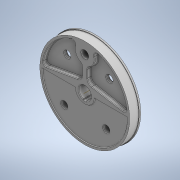
# Autodesk Inventor part: МТ10-3.00.00.02
Saved by Autodesk Inventor 2021 (Build 250183000, 183)
## iProperties
Created: 2022-06-08
Part Number: МТ10-3.00.00.02
Material: Типовые
Document SubType Name: Modeling
Designer: u
Density: 1 g/cm^3
Appearance: По умолчанию
Description: Диск
Mass: 2664.31 g
Surface Area: 2672.83 cm^2
Volume: 2664.31 cm^3
Author: u
Title: Диск
Autodesk Inventor part; units mm, degrees
ref_plane "YZ Plane" through (0, 0, 0) normal (1, 0, 0) x (0, 1, 0)
ref_plane "XZ Plane" through (0, 0, 0) normal (0, 1, 0) x (-1, 0, 0)
ref_plane "XY Plane" through (0, 0, 0) normal (0, 0, 1) x (1, 0, 0)
sketch "Эскиз1" plane through (0, 0, 0) normal (0, 0, 1) x (1, 0, 0)
  circle A0 centre (0, 0) radius 172
  circle A1 centre (0, 0) radius 162
  arc A2 (-36.4522, 138.735) -> (36.4522, 138.735) centre (0, 128) ccw
  arc A3 (-36.4522, 138.735) -> (-51.8004, 153.495) centre (-47.9634, 142.125) ccw
  circle A4 centre (0, 0) radius 38
  line L0 (26.527, 33.9088) -> (145.8715, 12.8651)
  line L1 (-240.8, 0) -> (240.8, 0) projected
  arc A5 (145.8715, 12.8651) -> (159.7917, 26.6575) centre (147.9553, 24.6828) ccw
  arc A6 (10, 53.6049) -> (26.527, 33.9088) centre (30, 53.6049) ccw
  line L2 (10, 53.6049) -> (10, 83.1001)
  arc A7 (16.72, 93.8761) -> (10, 83.1001) centre (22, 83.1001) ccw
  arc A8 (51.8004, 153.495) -> (36.4522, 138.735) centre (47.9634, 142.125) ccw
  arc A9 (-159.7917, 26.6575) -> (-145.8715, 12.8651) centre (-147.9553, 24.6828) ccw
  line L3 (-145.8715, 12.8651) -> (-26.527, 33.9088)
  arc A10 (-26.527, 33.9088) -> (-10, 53.6049) centre (-30, 53.6049) ccw
  line L4 (-10, 53.6049) -> (-10, 83.1001)
  arc A11 (-10, 83.1001) -> (-16.72, 93.8761) centre (-22, 83.1001) ccw
  line L5 (0, 0) -> (-80.6102, 80.6102)
  line L6 (6.4, -23.1309) -> (6.4, -26.9)
  line L7 (6.4, -26.9) -> (-6.4, -26.9)
  line L8 (-6.4, -26.9) -> (-6.4, -23.1309)
  arc A12 (6.4, -23.1309) -> (-6.4, -23.1309) centre (0, 0) ccw
  point P0 (-80.6102, -80.6102)
  point P1 (80.6102, -80.6102)
  point P2 (80.6102, 80.6102)
  point P3 (0, -26.9)
  point P4 (162, 0)
  point P5 (38, 0)
  point P6 (-38, 0)
  point P7 (-162, 0)
  dimension "d1" = 344
  dimension "d7" = 324
  dimension "d10" = 38
  dimension "d12" = 12
  dimension "d14" = 76
  dimension "d15" = 10
  dimension "d16" = 12
  dimension "d20" = 20
  dimension "d27" = 10
  dimension "d28" = 29.4952
  dimension "d29" = 12
  dimension "d31" = 12
  dimension "d33" = 12
  dimension "d36" = 10
  dimension "d37" = 20
  dimension "d38" = 12
  dimension "d39" = 45
  dimension "d40" = 114
  dimension "d43" = 360
  dimension "d45" = 26.9
  dimension "d46" = 12.8
  dimension "d47" = 24
  dimension "d61" = 128
  constraints: 26 point on circle, 16 end point, 16 tangent, 13 centre point, 4 coincident, 4 horizontal alignment, 3 vertical, 2 vertical alignment, 1 midpoint, 1 parallel, 5 other
  measures "d1" diameter of A0
  measures "d7" diameter of A1
  measures "d10" radius of A2
  measures "d12" radius of A3
  measures "d14" diameter of A4
  measures "d15" angle of L1 L0
  measures "d16" radius of A5
  measures "d20" radius of A6
  measures "d27" distance from line of L5.start L2
  measures "d28" distance of L2.start L2.end
  measures "d29" radius of A7
  measures "d31" radius of A8
  measures "d33" radius of A9
  measures "d36" angle of L1 L3
  measures "d37" radius of A10
  measures "d38" radius of A11
  measures "d39" angle of L1 L5
  measures "d40" distance of L5.start L5.end
  measures "d45" distance between parallel lines of L1 L7
  measures "d46" distance of L6.end L7.end
  measures "d47" radius of A12
  measures "d61" distance of L5.start A2.centre
extrude "Выдавливание1" add sketch "Эскиз1" along normal mid plane 12 contours A5 L0 A6 L2 A7 A2 A8 A1 | A1 A3 A2 A11 L4 A10 L3 A9
extrude "Выдавливание2" add sketch "Эскиз1" along normal mid plane 36 contours A1 L1 A4
extrude "Выдавливание3" add sketch "Эскиз1" along normal mid plane 40 contours L1 A1 A0 | A0 L1 A1 | L1 A4 L5 L3 A10 L4 A11 A2 A7 L2 A6 L0 A5 A1 | A1 A9 L3 L5 A4 L1 | L1 A12 L5 A4 | A4 L1 A12 L8 L7 L6 | A4 L5 A12 L1 | A8 A2 A3 A1
hole "Отверстие2" at (-80.6102, 80.6102, 0) at (-80.6102, -80.6102, 0) at (80.6102, -80.6102, 0) at (80.6102, 80.6102, 0) direction (0, 0, -1) diameter 24 end through all both
sketch "Эскиз2" plane through (0, 0, 20) normal (0, 0, 1) x (1, 0, 0)
  arc A0 (16.72, 93.8761) -> (36.4522, 138.735) centre (0, 128) ccw projected
  point P0 (0, 0)
  constraints: 1 coincident
hole "Отверстие3" at (0, 128, 20) direction (0, 0, -1) diameter 30 end through all
sketch "Эскиз4" plane through (0, 0, 0) normal (1, 0, 0) x (0, 1, 0)
  line L0 (172, -20) -> (172, 20) projected
  line L1 (172, -14) -> (174.5, -14)
  line L2 (174.5, -14) -> (174.5, -20)
  line L3 (174.5, -20) -> (172, -20)
  line L4 (0, 5.1312) -> (0, -5.1312)
  point P0 (0, 0)
  point P1 (0, 0)
  dimension "d80" = 2.5
  dimension "d81" = 6
  dimension "d82" = 10.2624
  constraints: 8 end point, 2 perpendicular, 1 coincident, 1 horizontal, 1 midpoint, 1 point on line, 1 vertical
  measures "d80" distance of L1.start L1.end
  measures "d81" distance of L1.end L2.end
  measures "d82" distance of L4.start L4.end
revolve "Вращение1" add sketch "Эскиз4" angle 360 about axis through (0, 0, 5.1312) along (0, 0, -1)
fillet "Сопряжение3" radius 2 72 edges at (-10, 68.3525, 6) (-11.8177, 89.4499, 6) (-34.7836, 112.6997, 6) (-39.6455, 150.7744, 6) (-123.3481, 105.0203, 6) (-156.4013, 16.1585, 6) (-86.1993, 23.387, 6) (-14.6791, 40.7492, 6) (-86.1993, 23.387, 20) (-156.4013, 16.1585, 20) (-123.3481, 105.0203, 20) (-39.6455, 150.7744, 20) (-34.7836, 112.6997, 20) (-11.8177, 89.4499, 20) (-10, 68.3525, 20) (-14.6791, 40.7492, 20) (10, 68.3525, 20) (11.8177, 89.4499, 20) (34.7836, 112.6997, 20) (39.6455, 150.7744, 20) (123.3481, 105.0203, 20) (156.4013, 16.1585, 20) (86.1993, 23.387, 20) (14.6791, 40.7492, 20) (39.6455, 150.7744, 6) (34.7836, 112.6997, 6) (11.8177, 89.4499, 6) (10, 68.3525, 6) (14.6791, 40.7492, 6) (86.1993, 23.387, 6) (156.4013, 16.1585, 6) (123.3481, 105.0203, 6) (0, -38, 20) (0, -162, 20) (100, 0, 20) (-100, 0, 20) (-100, 0, -20) (0, -38, -20) (100, 0, -20) (0, -162, -20) (39.6455, 150.7744, -20) (34.7836, 112.6997, -20) (11.8177, 89.4499, -20) (10, 68.3525, -20) (14.6791, 40.7492, -20) (86.1993, 23.387, -20) (156.4013, 16.1585, -20) (123.3481, 105.0203, -20) (-11.8177, 89.4499, -20) (-34.7836, 112.6997, -20) (-39.6455, 150.7744, -20) (-123.3481, 105.0203, -20) (-156.4013, 16.1585, -20) (-86.1993, 23.387, -20) (-14.6791, 40.7492, -20) (-10, 68.3525, -20) (-14.6791, 40.7492, -6) (-86.1993, 23.387, -6) (-156.4013, 16.1585, -6) (-123.3481, 105.0203, -6) (-39.6455, 150.7744, -6) (-34.7836, 112.6997, -6) (-11.8177, 89.4499, -6) (-10, 68.3525, -6) (14.6791, 40.7492, -6) (10, 68.3525, -6) (11.8177, 89.4499, -6) (34.7836, 112.6997, -6) (39.6455, 150.7744, -6) (123.3481, 105.0203, -6) (156.4013, 16.1585, -6) (86.1993, 23.387, -6)
sketch "Эскиз6" plane through (0, 0, -20) normal (0, 0, -1) x (-1, 0, 0)
  circle A0 centre (0, 128) radius 15 projected
  circle A1 centre (0, 128) radius 18
  point P0 (0, 0)
  dimension "d89" = 36
  constraints: 1 centre point, 1 coincident
  measures "d89" diameter of A1
extrude "Выдавливание4" cut sketch "Эскиз6" against normal blind 3.2
chamfer "Фаска3" distance 2 angle 45 11 edges at (0, 143, -16.8) (80.6102, 92.6102, -6) (80.6102, 92.6102, 6) (-80.6102, 92.6102, -6) (-80.6102, 92.6102, 6) (0, 24, -20) (0, 24, 20) (80.6102, -68.6102, -18) (80.6102, -68.6102, 18) (-80.6102, -68.6102, -18) (-80.6102, -68.6102, 18)
